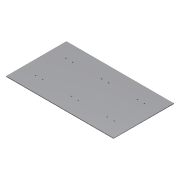
# Autodesk Inventor part: huta
Saved by Autodesk Inventor 2011 SP1 (Build 150282100, 282)
## iProperties
Created: 2012-11-12
Part Number: huta
Document SubType Name: Modeling
Designer: arihon
Density: 1 g/cm^3
Author: arihon
Autodesk Inventor part; units mm, degrees
ref_plane "YZ Plane" through (0, 0, 0) normal (1, 0, 0) x (0, 1, 0)
ref_plane "XZ Plane" through (0, 0, 0) normal (0, 1, 0) x (-1, 0, 0)
ref_plane "XY Plane" through (0, 0, 0) normal (0, 0, 1) x (1, 0, 0)
sketch "スケッチ1" plane through (0, 0, 0) normal (0, 0, 1) x (1, 0, 0)
  line L0 (-147, 82.5) -> (147, 82.5)
  line L1 (147, 82.5) -> (147, -82.5)
  line L2 (147, -82.5) -> (-147, -82.5)
  line L3 (-147, -82.5) -> (-147, 82.5)
  point P0 (0, 0)
  dimension "d0" = 294
  dimension "d1" = 165
  dimension "d2" = 147
  dimension "d3" = 82.5
  constraints: 8 end point, 2 parallel, 1 horizontal, 1 perpendicular
  measures "d0" distance of L1.end L2.end
  measures "d1" distance of L2.end L0.start
  measures "d2" distance from line of L3 point (0, 0)
  measures "d3" distance from line of point (0, 0) L0
extrude "押し出し1" add sketch "スケッチ1" along normal blind 2
sketch "スケッチ2" plane through (0, 0, 2) normal (0, 0, 1) x (1, 0, 0)
  line L0 (147, 82.5) -> (147, -82.5) projected
  line L1 (-147, 82.5) -> (147, 82.5) projected
  line L2 (-147, -82.5) -> (-147, 82.5) projected
  line L3 (147, -82.5) -> (-147, -82.5) projected
  line L4 (-147, -82.5) -> (-147, 82.5) projected
  line L5 (-147, 0) -> (147, 0)
  line L6 (-147, 41.25) -> (147, 41.25)
  line L7 (147, -41.25) -> (-147, -41.25)
  line L8 (0, 82.5) -> (0, -82.5)
  line L9 (-98, 82.5) -> (-98, -82.5)
  line L10 (98, 82.5) -> (98, -82.5)
  point P0 (0, 0)
  point P1 (-107.5, 41.25)
  point P2 (-88.5, 41.25)
  point P3 (-9.5, 41.25)
  point P4 (9.5, 41.25)
  point P5 (88.5, 41.25)
  point P6 (107.5, 41.25)
  point P7 (107.5, -41.25)
  point P8 (88.5, -41.25)
  point P9 (9.5, -41.25)
  point P10 (-9.5, -41.25)
  point P11 (-88.5, -41.25)
  point P12 (-107.5, -41.25)
  dimension "d6" = 41.25
  dimension "d7" = 41.25
  dimension "d8" = 98
  dimension "d9" = 98
  dimension "d22" = 19
  dimension "d23" = 9.5
  dimension "d24" = 19
  dimension "d25" = 9.5
  dimension "d26" = 19
  dimension "d27" = 9.5
  dimension "d28" = 19
  dimension "d29" = 9.5
  dimension "d30" = 19
  dimension "d31" = 9.5
  dimension "d32" = 19
  dimension "d33" = 9.5
  constraints: 20 point on line, 12 end point, 4 midpoint, 3 perpendicular, 1 parallel
  measures "d6" distance between parallel lines of L6 L1
  measures "d7" distance between parallel lines of L3 L7
  measures "d8" distance between parallel lines of L8 L9
  measures "d9" distance between parallel lines of L8 L10
  measures "d22" distance of point (-88.5, 41.25) point (-107.5, 41.25)
  measures "d23" distance from line of L9 point (-88.5, 41.25)
  measures "d24" distance of point (9.5, 41.25) point (-9.5, 41.25)
  measures "d25" distance from line of L8 point (9.5, 41.25)
  measures "d26" distance of point (107.5, 41.25) point (88.5, 41.25)
  measures "d27" distance from line of L10 point (107.5, 41.25)
  measures "d28" distance of point (-107.5, -41.25) point (-88.5, -41.25)
  measures "d29" distance from line of point (-88.5, -41.25) L9
  measures "d30" distance of point (9.5, -41.25) point (-9.5, -41.25)
  measures "d31" distance from line of point (9.5, -41.25) L8
  measures "d32" distance of point (107.5, -41.25) point (88.5, -41.25)
  measures "d33" distance from line of L10 point (107.5, -41.25)
hole "Hole1" at (-107.5, 41.25, 2) at (-88.5, 41.25, 2) at (-9.5, 41.25, 2) at (9.5, 41.25, 2) at (88.5, 41.25, 2) at (107.5, 41.25, 2) at (107.5, -41.25, 2) at (88.5, -41.25, 2) at (9.5, -41.25, 2) at (-9.5, -41.25, 2) at (-88.5, -41.25, 2) at (-107.5, -41.25, 2) direction (0, 0, -1) diameter 3.2 end through all
equation "\"d2\" = 0.5 * d0"
equation "\"d3\" = 0.5 * d1"
equation "\"d7\" = d6"
equation "\"d9\" = d8"
equation "\"d23\" = 0.5 * d22"
equation "\"d24\" = d22"
equation "\"d25\" = d23"
equation "\"d26\" = d22"
equation "\"d27\" = d23"
equation "\"d28\" = d22"
equation "\"d29\" = d23"
equation "\"d30\" = d22"
equation "\"d31\" = d23"
equation "\"d32\" = d22"
equation "\"d33\" = d23"
